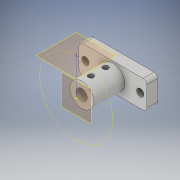
# Autodesk Inventor part: spannring_achse
Saved by Autodesk Inventor 2017 (Build 210142000, 142)
## iProperties
Part Number: spannring_achse
Material: Generisch
Document SubType Name: Modeling
Designer: Fabio
Density: 1 g/cm^3
Appearance: Vorgabe
Author: Fabio
Autodesk Inventor part; units mm, degrees
ref_plane "YZ Plane" through (0, 0, 0) normal (1, 0, 0) x (0, 1, 0)
ref_plane "XZ Plane" through (0, 0, 0) normal (0, 1, 0) x (-1, 0, 0)
ref_plane "XY Plane" through (0, 0, 0) normal (0, 0, 1) x (1, 0, 0)
sketch "Skizze1" plane through (0, 0, 0) normal (0, 1, 0) x (-1, 0, 0)
  circle A0 centre (0, 0) radius 20
  dimension "d0" = 40
  constraints: 1 centre point, 1 coincident
  measures "d0" diameter of A0
extrude "Extrusion1" add sketch "Skizze1" along normal blind 26
ref_plane "Arbeitsebene1" through (0, 26, 0) normal (0, 1, 0) x (1, 0, 0)
sketch "Skizze2" plane through (0, 26, 0) normal (0, 1, 0) x (1, 0, 0)
  circle A0 centre (0, 0) radius 20 projected
  circle A1 centre (0, 0) radius 20 construction
  circle A2 centre (0, 0) radius 20 construction
  line L0 (-15, 0) -> (15, 0) construction
  dimension "d42" = 15
  dimension "d43" = 15
  constraints: 2 coincident, 2 end point, 1 horizontal
  measures "d42" distance of point (0, 0) L0.start
  measures "d43" distance of point (0, 0) point (15, 0)
ref_plane "Arbeitsebene2" through (0, 0, 0) normal (0, -1, 0) x (1, 0, 0)
sketch "Skizze3" plane through (0, 0, 0) normal (0, -1, 0) x (1, 0, 0)
  circle A0 centre (0, 0) radius 20 projected
  constraints: 1 coincident
hole "Bohrung2" at (0, 0, 0) direction (0, 1, 0) diameter 6 depth 20
sketch "Skizze4" plane through (0, 0, 0) normal (0, -1, 0) x (1, 0, 0)
  point P0 (0, 0)
sketch "Skizze5" plane through (0, 0, 0) normal (0, -1, 0) x (1, 0, 0)
  line L0 (0, 0) -> (0, 20) construction
  circle A0 centre (0, 0) radius 20 construction
  constraints: 2 end point, 1 coincident, 1 vertical, 1 vertical alignment, 1 other
ref_plane "Arbeitsebene3" through (0, 0, 20) normal (0, 0, 1) x (1, 0, 0)
sketch "Skizze6" plane through (0, 0, 20) normal (0, 0, 1) x (1, 0, 0)
  line L0 (0, 0) -> (0, 27.6738) construction
  point P0 (0, 8)
  point P1 (0, 16)
  dimension "d25" = 8
  dimension "d26" = 8
  constraints: 2 end point, 2 point on line, 1 vertical
  measures "d25" distance of point (0, 16) point (0, 8)
  measures "d26" distance of L0.start point (0, 8)
hole "Bohrung3" at (0, 16, 20) at (0, 8, 20) direction (0, 0, -1) diameter 3 depth 20 tip angle 118
sketch "Skizze7" plane through (0, 0, 0) normal (0, -1, 0) x (1, 0, 0)
  circle A0 centre (0, 0) radius 6.5
  circle A1 centre (0, 0) radius 20
  dimension "d38" = 13
  dimension "d39" = 40
  constraints: 2 centre point, 2 coincident
  measures "d38" diameter of A0
  measures "d39" diameter of A1
extrude "Extrusion2" cut sketch "Skizze7" against normal blind 20
hole "Bohrung4" at (-15, 26, 0) at (15, 26, 0) direction (0, -1, 0) diameter 4 end through all
sketch "Skizze8" plane through (0, 0, 0) normal (0, -1, 0) x (1, 0, 0)
  line L0 (-20, 7.5) -> (20, 7.5)
  line L1 (20, 7.5) -> (20, -7.5)
  line L2 (20, -7.5) -> (-20, -7.5)
  line L3 (-20, -7.5) -> (-20, 7.5)
  line L4 (-20, 7.5) -> (20, -7.5) construction
  line L5 (20, 7.5) -> (-20, -7.5) construction
  point P0 (0, 0)
  dimension "d52" = 40
  dimension "d53" = 15
  constraints: 12 end point, 2 midpoint, 2 parallel, 1 horizontal, 1 perpendicular
  measures "d52" distance of L1.end L2.end
  measures "d53" distance of L0.end L1.end
extrude "Extrusion3" cut sketch "Skizze8" against normal through all keep common part
sketch "Skizze9" plane through (0, 0, 0) normal (0, -1, 0) x (1, 0, 0)
  line L0 (-15, -15) -> (15, -15)
  line L1 (15, -15) -> (15, 15)
  line L2 (15, 15) -> (-15, 15)
  line L3 (-15, 15) -> (-15, -15)
  line L4 (-15, -15) -> (15, 15) construction
  line L5 (15, -15) -> (-15, 15) construction
  point P0 (0, 0)
  dimension "d56" = 30
  dimension "d57" = 30
  constraints: 12 end point, 2 midpoint, 2 parallel, 1 horizontal, 1 perpendicular
  measures "d56" distance of L2.end L1.end
  measures "d57" distance of L1.end L0.end
extrude "Extrusion4" cut sketch "Skizze9" against normal blind 3
thread "Gewinde5" size "M3x0.5" class "6H" standard "ANSI Metric M Profile" full length
thread "Gewinde6" size "M3x0.5" class "6H" standard "ANSI Metric M Profile" full length
thread "Gewinde7" size "M4x0.7" class "6H" standard "ANSI Metric M Profile" full length
thread "Gewinde8" size "M4x0.7" class "6H" standard "ANSI Metric M Profile" full length
sketch "Skizze10" plane through (0, 26, 0) normal (0, 1, 0) x (1, 0, 0)
  arc A0 (-18.5405, 7.5) -> (-18.5405, -7.5) centre (0, 0) ccw projected
  line L0 (18.5405, 7.5) -> (-18.5405, 7.5)
  line L1 (-18.5405, 7.5) -> (-18.5405, -7.5)
  line L2 (-18.5405, -7.5) -> (18.5405, -7.5)
  line L3 (18.5405, -7.5) -> (18.5405, 7.5)
  line L4 (18.5405, 7.5) -> (-18.5405, -7.5) construction
  line L5 (-18.5405, 7.5) -> (18.5405, -7.5) construction
  constraints: 12 end point, 2 midpoint, 2 parallel, 1 horizontal, 1 perpendicular
extrude "Extrusion5" cut sketch "Skizze10" against normal through all contours L0 L3 L2 L1 keep common part
fillet "Rundung1" radius 2 4 edges at (18.5405, 23, -7.5) (18.5405, 23, 7.5) (-18.5405, 23, -7.5) (-18.5405, 23, 7.5)
